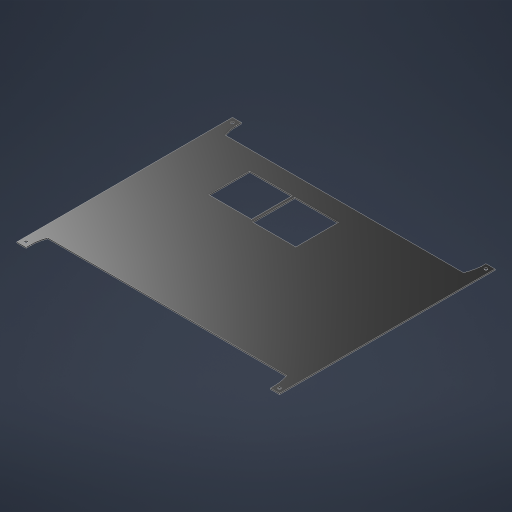
# Autodesk Inventor part: belly pan
Saved by Autodesk Inventor 2024 (Build 280153000, 153)
## iProperties
Created: 2023-12-20
Part Number: belly pan
Material: Generic
Document SubType Name: Modeling
Designer: elite
Density: 1 g/cm^3
Appearance: Glossy - Black
Author: elite
Autodesk Inventor part; units mm, degrees
ref_plane "YZ Plane" through (0, 0, 0) normal (1, 0, 0) x (0, 1, 0)
ref_plane "XZ Plane" through (0, 0, 0) normal (0, 1, 0) x (-1, 0, 0)
ref_plane "XY Plane" through (0, 0, 0) normal (0, 0, 1) x (1, 0, 0)
sketch "Sketch1" plane through (0, 0, 0) normal (0, 1, 0) x (-1, 0, 0)
  line L0 (0, 0) -> (355.6, 0)
  line L1 (355.6, 0) -> (355.6, -289.56)
  line L2 (355.6, -289.56) -> (0, -289.56)
  line L3 (0, -289.56) -> (0, 0)
  circle A0 centre (355.6, 0) radius 2.1082
  line L4 (355.6, 0) -> (361.95, 0)
  line L5 (355.6, 0) -> (355.6, 6.35)
  line L6 (355.6, 6.35) -> (361.95, 6.35)
  line L7 (0, -289.56) -> (0, -295.91)
  line L8 (0, -295.91) -> (-6.35, -295.91)
  line L9 (-6.35, -295.91) -> (361.95, -295.91)
  line L10 (361.95, -295.91) -> (361.95, 6.35)
  line L11 (361.95, 6.35) -> (-6.35, 6.35)
  line L12 (-6.35, 6.35) -> (-6.35, -295.91)
  circle A1 centre (355.6, -289.56) radius 2.1082
  circle A2 centre (0, -289.56) radius 2.1082
  circle A3 centre (0, 0) radius 2.1082
  line L13 (0, 0) -> (0, -20.32)
  line L14 (0, -20.32) -> (10.16, -20.32)
  line L15 (0, 0) -> (5.08, 0)
  line L16 (0, -289.56) -> (5.08, -289.56)
  line L17 (0, -289.56) -> (0, -269.24)
  line L18 (0, -269.24) -> (11.0826, -269.24)
  line L19 (355.6, 0) -> (355.6, -20.32)
  line L20 (355.6, -20.32) -> (345.44, -20.32)
  line L21 (355.6, 0) -> (350.52, 0)
  line L22 (355.6, -289.56) -> (350.52, -289.56)
  line L23 (355.6, -289.56) -> (355.6, -269.24)
  line L24 (355.6, -269.24) -> (345.44, -269.24)
  line L25 (345.44, -20.32) -> (10.16, -20.32)
  line L26 (355.6, -20.32) -> (355.6, -33.02)
  line L27 (355.6, -33.02) -> (0, -33.02)
  line L28 (355.6, -269.24) -> (355.6, -256.54)
  line L29 (355.6, -256.54) -> (0, -256.54)
  line L30 (345.44, -269.24) -> (11.0826, -269.24)
  line L31 (0, 0) -> (6.35, 0)
  arc A4 (6.35, 0) -> (10.16, -20.32) centre (82.4575, 3.753) ccw
  line L32 (6.35, 0) -> (-6.35, 0)
  line L33 (-6.35, 0) -> (-6.35, -289.56)
  line L34 (-6.35, -289.56) -> (6.35, -289.56)
  line L35 (6.35, -289.56) -> (6.35, 0)
  arc A5 (11.0826, -269.24) -> (6.35, -289.56) centre (82.2313, -296.5221) ccw
  line L36 (355.6, 0) -> (349.25, 0)
  line L37 (349.25, 0) -> (349.25, -289.56)
  arc A6 (349.25, -289.56) -> (345.44, -269.24) centre (298.4597, -288.566) ccw
  arc A7 (345.44, -20.32) -> (349.25, 0) centre (298.4597, -0.994) ccw
  line L38 (349.25, 0) -> (349.25, 6.35)
  line L39 (349.25, -289.56) -> (349.25, -295.91)
  line L40 (6.35, -289.56) -> (6.35, -295.91)
  line L41 (6.35, 0) -> (6.35, 6.35)
  dimension "d0" = 355.6
  dimension "d1" = 289.56
  dimension "d2" = 4.2164
  dimension "d3" = 6.35
  dimension "d4" = 6.35
  dimension "d5" = 6.35
  dimension "d6" = 6.35
  dimension "d7" = 20.32
  dimension "d8" = 10.16
  dimension "d10" = 20.32
  dimension "d12" = 20.32
  dimension "d13" = 10.16
  dimension "d16" = 5.08
  dimension "d17" = 20.32
  dimension "d18" = 10.16
  dimension "d20" = 12.7
  dimension "d21" = 12.7
  dimension "d23" = 6.35
  dimension "d24" = 76.2
  dimension "d25" = 76.2
  dimension "d26" = 6.35
  dimension "d27" = 50.8
  dimension "d28" = 50.8
  constraints: 84 end point, 21 point on line, 14 perpendicular, 8 centre point, 8 point on circle, 6 parallel, 5 horizontal, 4 coincident, 2 vertical
  measures "d0" distance of L1.end L2.end
  measures "d1" distance of L2.end L0.start
  measures "d2" diameter of A0
  measures "d3" distance of L4.start L4.end
  measures "d4" distance of L4.start L5.end
  measures "d5" distance of L2.end L7.end
  measures "d6" distance of L7.end L8.end
  measures "d7" distance of L13.start L13.end
  measures "d8" distance of L13.end L14.end
  measures "d10" distance of L16.start L17.end
  measures "d12" distance of L4.start L19.end
  measures "d13" distance of L19.end L20.end
  measures "d16" distance of L22.start L22.end
  measures "d17" distance of L22.start L23.end
  measures "d18" distance of L23.end L24.end
  measures "d20" distance of L19.end L26.end
  measures "d21" distance of L23.end L28.end
  measures "d23" distance of L13.start L31.end
  measures "d24" radius of A4
  measures "d25" radius of A5
  measures "d26" distance of L4.start L36.end
  measures "d27" radius of A6
  measures "d28" radius of A7
extrude "Extrusion1" add sketch "Sketch1" along normal blind 1.5875 contours A3 L32 L12 L11 L41 L0 | L0 L35 L14 L3 A3 | L3 A2 L34 L12 L32 A3 | L14 L35 L27 L3 | A4 L14 L35 | L27 L35 L29 L3 | L14 L25 L20 L37 L27 L35 | L34 A2 L7 L8 L12 | L38 L11 L5 A0 L0 | L0 A0 L1 L20 L37 A7 | L29 L35 L18 L3 | L27 L37 L29 L35 | L37 L20 A7 | L18 L35 L2 A2 L3 | L29 L37 L24 L30 L18 L35 | L37 L20 L1 L27 | L27 L1 L29 L37 | L7 A2 L2 L40 L9 | L6 L10 L4 A0 L5 | L18 A5 L35 | L29 L1 L24 L37 | L1 A0 L4 L10 L9 L39 L2 A1 | L37 A6 L24 | L24 L1 A1 L2 A6 L37
sketch "Sketch2" plane through (0, 1.5875, 0) normal (0, 1, 0) x (1, 0, 0)
  circle A0 centre (-355.6, 289.56) radius 2.1082 projected
  line L0 (-355.6, 289.56) -> (-355.6, 248.412)
  line L1 (-355.6, 248.412) -> (-284.48, 248.412)
  line L2 (-355.6, 289.56) -> (-355.6, 185.42)
  line L3 (-355.6, 185.42) -> (-224.79, 185.42)
  line L4 (-284.48, 248.412) -> (-224.79, 248.412)
  line L5 (-224.79, 248.412) -> (-224.79, 185.42)
  line L6 (-224.79, 185.42) -> (-284.48, 185.42)
  line L7 (-284.48, 185.42) -> (-284.48, 248.412)
  line L8 (-355.6, 289.56) -> (-355.6, 242.57)
  line L9 (-355.6, 242.57) -> (-220.98, 242.57)
  line L10 (-355.6, 289.56) -> (-355.6, 184.15)
  line L11 (-355.6, 289.56) -> (-355.6, 182.88)
  line L12 (-355.6, 182.88) -> (-160.02, 182.88)
  line L13 (-220.98, 242.57) -> (-160.02, 242.57)
  line L14 (-160.02, 242.57) -> (-160.02, 182.88)
  line L15 (-160.02, 182.88) -> (-220.98, 182.88)
  line L16 (-220.98, 182.88) -> (-220.98, 242.57)
  point P0 (0, 0)
  point P1 (-224.79, 242.57)
  point P2 (-284.48, 242.57)
  dimension "d31" = 41.148
  dimension "d32" = 71.12
  dimension "d33" = 104.14
  dimension "d34" = 130.81
  dimension "d35" = 46.99
  dimension "d36" = 134.62
  dimension "d37" = 105.41
  dimension "d38" = 106.68
  dimension "d39" = 195.58
  constraints: 34 end point, 5 parallel, 5 perpendicular, 4 point on line, 2 horizontal, 1 vertical
  measures "d31" distance of L0.start L0.end
  measures "d32" distance of L0.end L1.end
  measures "d33" distance of L0.start L2.end
  measures "d34" distance of L2.end L3.end
  measures "d35" distance of L0.start L8.end
  measures "d36" distance of L8.end L9.end
  measures "d37" distance of L0.start L10.end
  measures "d38" distance of L0.start L11.end
  measures "d39" distance of L11.end L12.end
extrude "Extrusion2" cut sketch "Sketch2" against normal blind 25.4 contours L9 L5 L3 L7 | L13 L14 L12 L16
body "Solid1"
